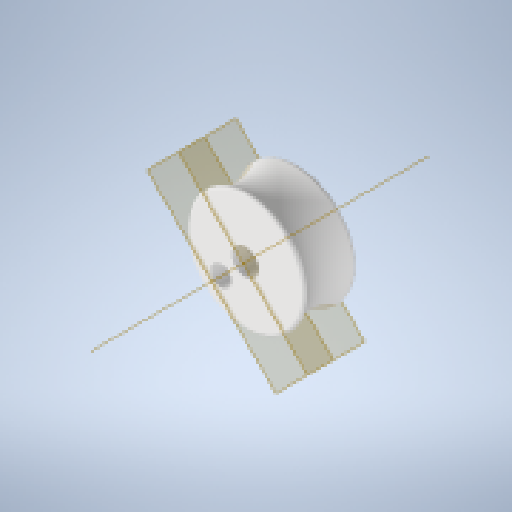
# Autodesk Inventor part: StringPulley
Saved by Autodesk Inventor 2023 (Build 270158000, 158)
## iProperties
Created: 2023-09-03
Part Number: StringPulley
Material: Generic
Document SubType Name: Modeling
Designer: Felix
Density: 1 g/cm^3
Appearance: Default
Author: Felix
Autodesk Inventor part; units mm, degrees
ref_plane "YZ Plane" through (0, 0, 0) normal (1, 0, 0) x (0, 1, 0)
ref_plane "XZ Plane" through (0, 0, 0) normal (0, 1, 0) x (-1, 0, 0)
ref_plane "XY Plane" through (0, 0, 0) normal (0, 0, 1) x (1, 0, 0)
sketch "Sketch1" plane through (0, 0, 0) normal (0, 1, 0) x (-1, 0, 0)
  line L0 (0, 0) -> (10.7058, 0)
  line L1 (10.7058, 10) -> (0, 10)
  line L2 (0, 10) -> (0, 0)
  arc A0 (11.1388, 9.25) -> (11.1388, 0.75) centre (18.5, 5) ccw
  arc A1 (11.1388, 9.25) -> (10.7058, 10) centre (10.7058, 9.5) ccw
  arc A2 (10.7058, 0) -> (11.1388, 0.75) centre (10.7058, 0.5) ccw
  point P0 (10, 5)
  dimension "d1" = 10
  dimension "d3" = 0.5
  dimension "d5" = 10
  dimension "d24" = 60
  constraints: 7 point on circle, 6 end point, 4 tangent, 3 centre point, 1 equal radius, 1 horizontal, 1 parallel, 1 perpendicular, 1 vertical alignment
  measures "d1" distance of L1.end L0.start
  measures "d3" radius of A1
  measures "d5" distance from line of point (10, 5) L2
revolve "Revolution1" add sketch "Sketch1" angle 360 about axis through (0, 0, 10) along (0, 0, -1)
sketch "Sketch2" plane through (0, 0, 10) normal (0, 0, 1) x (1, 0, 0)
  point P0 (0, 0)
hole "Hole1" at (0, 0, 10) direction (0, 0, -1) diameter 5.1 end through all clearance for "Countersunk Flat Head Screw DIN EN ISO 2009" size "M5" standard "DIN"
sketch "Sketch3" plane through (0, 0, 0) normal (1, 0, 0) x (0, 1, 0)
  line L0 (-11.1388, 9.25) -> (11.1388, 9.25) construction
  line L1 (-11.1388, 0.75) -> (11.1388, 0.75) construction
  line L2 (-11.1388, 0.75) -> (11.1388, 0.75) construction
  line L3 (0, 0.75) -> (0, 9.25) construction
  line L4 (-11.1388, 9.25) -> (11.1388, 9.25) construction
  point P0 (0, 0)
  point P1 (0, 5)
  constraints: 3 midpoint, 2 end point
hole "Hole2" at (0, 0, 5) direction (-1, 0, 0) diameter 4.3 end through all
sketch "Sketch7" plane through (0, 0, 0) normal (0, 0, -1) x (-1, 0, 0)
  circle A0 centre (0, 0) radius 2.55 construction
  circle A1 centre (0, 0) radius 2.55 construction
  circle A2 centre (0, 0) radius 11.1388 construction
  circle A3 centre (0, 0) radius 10.7058 construction
  circle A4 centre (0, 0) radius 2.55 construction
  line L0 (0, 0) -> (7.8763, -7.8763) construction
  line L1 (0, 0) -> (10.2764, 0) construction
  point P0 (1.3711, 2.15)
  point P1 (1.3711, 2.15)
  point P2 (4.5962, -4.5962)
  dimension "d51" = 45
  dimension "d52" = 6.5
  constraints: 4 end point, 1 horizontal, 1 point on line, 2 other
  measures "d51" angle of L1 L0
  measures "d52" distance of A0.centre point (4.596, -4.596)
hole "Hole6" at (-4.5962, -4.5962, 0) direction (0, 0, 1) diameter 4 end through all
ref_plane "Work Plane4" through (-6.0104, -6.0104, 33.2348) normal (0.7071068, 0.7071068, 0) x (0, 0, 1)
ref_plane "Work Plane3" through (0, 0, -23.2348) normal (0.7071068, 0.7071068, 0) x (0, 0, 1)
sketch "Sketch8" plane through (-6.0104, -6.0104, 33.2348) normal (0.7071068, 0.7071068, 0) x (0, 0, 1)
  line L0 (-23.2348, 2) -> (-23.2348, -2) construction
  line L1 (-33.2348, -2) -> (-33.2348, 2) construction
  line L2 (-23.2348, 2) -> (-23.2348, -2) construction
  line L3 (-23.2348, 0) -> (-33.2348, 0) construction
  point P0 (-28.2348, 0)
  constraints: 2 end point, 2 midpoint, 1 horizontal
hole "Hole7" at (-6.0104, -6.0104, 5) direction (-0.7071068, -0.7071068, 0) diameter 2 end through all
hole "Hole8" at (-6.0104, -6.0104, 5) direction (0.7071068, 0.7071068, 0) diameter 2 end up to surface
ref_plane "Work Plane2" through (0, 0, -23.2348) normal (0.7071068, -0.7071068, 0) x (0, 0, 1)
body "Solid1"
